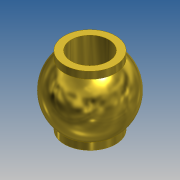
# Autodesk Inventor part: Boule_tete_verin
Saved by Autodesk Inventor 2021.3 (Build 253353000, 353)
## iProperties
Created: 2023-04-12
Part Number: Boule_tete_verin
Material: Copper, Alloy
Document SubType Name: Modeling
Designer: cedric.clivaz
Density: 8.92 g/cm^3
Appearance: Metal 2400F Hot
Author: cedric.clivaz
Autodesk Inventor part; units mm, degrees
ref_plane "YZ Plane" through (0, 0, 0) normal (1, 0, 0) x (0, 1, 0)
ref_plane "XZ Plane" through (0, 0, 0) normal (0, 1, 0) x (-1, 0, 0)
sketch "Sketch2" plane through (0, 0, 0) normal (0, 0, 1) x (1, 0, 0)
  line L0 (-4.2, 0) -> (4.2, 0) construction
  line L1 (0, -4.2) -> (0, 4.2) construction
  circle A0 centre (0, 0) radius 3
  line L2 (-3, 0) -> (3, 0)
  dimension "d0" = 6
  constraints: 2 end point, 2 point on circle, 2 point on line, 1 centre point, 1 coincident
  measures "d0" diameter of A0
revolve "Revolution1" add sketch "Sketch2" angle 360 about axis through (-10, 0, 0) along (1, 0, 0) picked at (0.7485, 0.6631) contours L2 A0
sketch "Sketch3" plane through (0, 0, 0) normal (0, 0, 1) x (1, 0, 0)
  circle A0 centre (0, 0) radius 1.5
  dimension "d2" = 3
  constraints: 1 centre point, 1 coincident
  measures "d2" diameter of A0
extrude "Extrusion1" cut sketch "Sketch3" along normal through all both and the other way through all
ref_plane "Work Plane1" through (0, 0, 2.75) normal (0, 0, 1) x (1, 0, 0)
sketch "Sketch4" plane through (0, 0, 2.75) normal (0, 0, 1) x (1, 0, 0)
  circle A0 centre (0, 0) radius 1.5 construction
  circle A1 centre (0, 0) radius 1.5
  circle A2 centre (0, 0) radius 2.05
  dimension "d6" = 4.1
  constraints: 2 centre point, 2 coincident, 1 concentric
  measures "d6" diameter of A2
extrude "Extrusion2" add sketch "Sketch4" against normal up to surface
mirror "Mirror1" about plane through (0, 0, 0) normal (0, 0, 1) of "Extrusion2"
body "Solid1"
